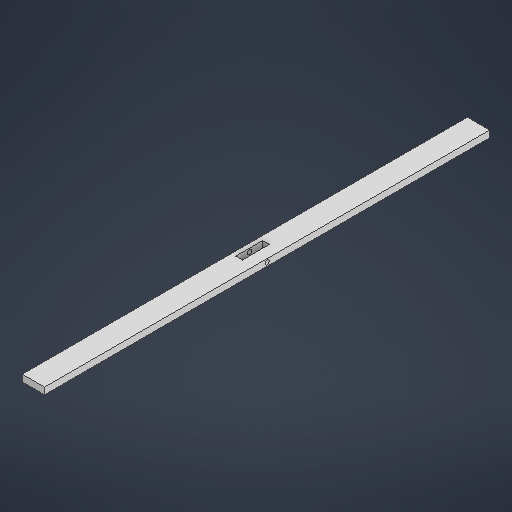
# Autodesk Inventor part: Layer
Saved by Autodesk Inventor 2026.1 (Build 301233020, 233B)
## iProperties
Created: 2026-03-11
Part Number: Layer
Material: Generic
Document SubType Name: Modeling
Designer: elaij
Density: 1 g/cm^3
Appearance: Default
Author: elaij
Autodesk Inventor part; units mm, degrees
ref_plane "YZ Plane" through (0, 0, 0) normal (1, 0, 0) x (0, 1, 0)
ref_plane "XZ Plane" through (0, 0, 0) normal (0, 1, 0) x (-1, 0, 0)
ref_plane "XY Plane" through (0, 0, 0) normal (0, 0, 1) x (1, 0, 0)
sketch "Sketch1" plane through (0, 0, 0) normal (0, 0, 1) x (1, 0, 0)
  line L0 (-25, 7.5) -> (25, 7.5)
  line L1 (25, 7.5) -> (25, -7.5)
  line L2 (25, -7.5) -> (-25, -7.5)
  line L3 (-25, -7.5) -> (-25, 7.5)
  line L4 (0, 0) -> (0, 14.2686)
  line L5 (0, 0) -> (7.5147, 0)
  dimension "d2" = 50
  dimension "d3" = 15
  constraints: 12 end point, 2 horizontal, 2 parallel, 1 perpendicular, 1 vertical, 2 other
  measures "d2" distance between parallel lines of L1 L3
  measures "d3" distance between parallel lines of L0 L2
extrude "Extrusion1" add sketch "Sketch1" along normal blind 1000
sketch "Sketch4" plane through (-25, 7.5, 0) normal (0, 1, 0) x (1, 0, 0)
  line L0 (25, 0) -> (25, -1000)
  line L1 (0, -1000) -> (50, -1000) projected
  line L2 (0, 0) -> (0, -1000) projected
  line L3 (0, -500) -> (50, -500)
  line L4 (50, 0) -> (50, -1000) projected
  line L5 (25, -530) -> (10, -530)
  line L6 (10, -530) -> (10, -470)
  line L7 (10, -470) -> (25, -470)
  line L8 (25, -470) -> (25, -530)
  dimension "d14" = 15
  dimension "d15" = 60
  constraints: 12 end point, 3 midpoint, 2 parallel, 1 horizontal, 1 perpendicular, 1 point on line, 1 other
  measures "d14" distance between parallel lines of L0 L6
  measures "d15" distance between parallel lines of L5 L7
extrude "Extrusion4" cut sketch "Sketch4" against normal through all contours L5 L6 L3 L0 | L3 L6 L7 L0
sketch "Sketch5" plane through (0, 7.5, 470) normal (-1, 0, 0) x (0, 0, 1)
  line L0 (0, 0) -> (60, 0) projected
  line L1 (30, 0) -> (30, -15)
  line L2 (60, -15) -> (0, -15) projected
  line L3 (60, 0) -> (60, -15) projected
  line L4 (60, -7.5) -> (0, -7.5)
  line L5 (0, 0) -> (0, -15) projected
  circle A0 centre (30, -7.5) radius 5
  point P0 (-470, -7.5)
  dimension "d18" = 10
  constraints: 5 midpoint, 4 end point, 1 centre point
  measures "d18" diameter of A0
extrude "Extrusion5" cut sketch "Sketch5" along normal through all both and the other way through all contours A0 L4 L1 | L1 L4 A0 | L4 L1 A0 | L4 A0 L1
body "Solid1"
